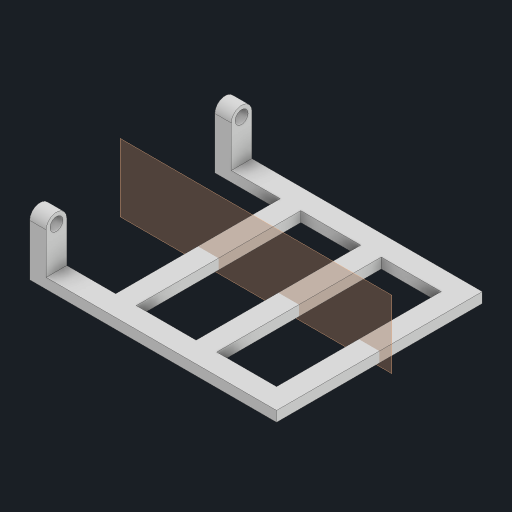
# Autodesk Inventor part: table_base
Saved by Autodesk Inventor 2024 (Build 280153000, 153)
## iProperties
Created: 2024-06-21
Part Number: table_base
Material: Generic
Document SubType Name: Modeling
Designer: mihir
Density: 1 g/cm^3
Appearance: Default
Author: mihir
Autodesk Inventor part; units mm, degrees
ref_plane "YZ Plane" through (0, 0, 0) normal (1, 0, 0) x (0, 1, 0)
ref_plane "XZ Plane" through (0, 0, 0) normal (0, 1, 0) x (-1, 0, 0)
ref_plane "XY Plane" through (0, 0, 0) normal (0, 0, 1) x (1, 0, 0)
sketch "Sketch1" plane through (0, 0, 0) normal (0, 1, 0) x (-1, 0, 0)
  line L0 (0, 0) -> (0, -100)
  line L1 (0, -100) -> (120, -100)
  line L2 (120, -100) -> (120, -90)
  line L3 (120, -90) -> (88.2057, -90)
  line L4 (88.2057, -90) -> (88.2057, -10)
  line L5 (88.2057, -10) -> (120, -10)
  line L6 (120, -10) -> (120, 0)
  line L7 (120, 0) -> (0, 0)
  line L8 (78.2057, -10) -> (49.1029, -10)
  line L9 (49.1029, -10) -> (49.1029, -90)
  line L10 (49.1029, -90) -> (78.2057, -90)
  line L11 (78.2057, -90) -> (78.2057, -10)
  line L12 (39.1029, -10) -> (10, -10)
  line L13 (10, -10) -> (10, -90)
  line L14 (10, -90) -> (39.1029, -90)
  line L15 (39.1029, -90) -> (39.1029, -10)
  dimension "d0" = 29.1029
  dimension "d1" = 120
  dimension "d2" = 10
  dimension "d3" = 100
  dimension "d4" = 10
  dimension "d5" = 10
  dimension "d6" = 10
  constraints: 32 end point, 8 perpendicular, 4 parallel, 4 point on line, 3 equal length, 2 horizontal, 1 collinear, 1 vertical
  measures "d0" distance of L13.end L14.end
  measures "d1" distance of L0.end L1.end
  measures "d2" distance of L5.end L6.end
  measures "d3" distance of L0.start L0.end
  measures "d4" distance between parallel lines of L4 L11
  measures "d5" distance between parallel lines of L0 L13
  measures "d6" distance between parallel lines of L9 L15
extrude "Extrusion1" add sketch "Sketch1" along normal blind 5
sketch "Sketch2" plane through (-120, 0, -10) normal (-1, 0, 0) x (0, 0, 1)
  line L0 (0, 0) -> (0, 5) projected
  line L1 (0, 0) -> (10, 0)
  line L2 (10, 0) -> (10, 25)
  line L3 (10, 25) -> (0, 25)
  line L4 (0, 25) -> (0, 0)
  circle A0 centre (5, 25) radius 3.15
  arc A1 (10, 25) -> (0, 25) centre (5, 25) ccw
  line L5 (10, 0) -> (10, 5) projected
  dimension "d9" = 25
  dimension "d10" = 6.3
  constraints: 8 end point, 2 centre point, 2 parallel, 2 point on circle, 1 coincident, 1 collinear, 1 horizontal, 1 midpoint, 1 perpendicular
  measures "d9" distance of L1.end L2.end
  measures "d10" diameter of A0
extrude "Extrusion2" add sketch "Sketch2" against normal blind 8
sketch "Sketch3" plane through (-112, 0, -10) normal (1, 0, 0) x (0, 0, -1)
  arc A0 (0, 25) -> (-10, 25) centre (-5, 25) ccw projected
  circle A1 centre (-5, 25) radius 3.15
  point P0 (-10, 0)
  dimension "d13" = 6.3
  constraints: 1 centre point, 1 coincident
  measures "d13" diameter of A1
extrude "Extrusion3" cut sketch "Sketch3" against normal blind 6
ref_plane "Work Plane1" through (-120, 0, -50) normal (0, 0, 1) x (1, 0, 0)
mirror "Mirror1" about plane through (-120, 0, -50) normal (0, 0, 1) of "Extrusion2", "Extrusion3"
equation "\"d1\" = table_base_length"
equation "\"d2\" = table_base_web_width"
equation "\"d3\" = table_base_width"
equation "\"d4\" = table_base_web_width"
equation "\"d5\" = table_base_web_width"
equation "\"d6\" = table_base_web_width"
equation "\"d7\" = table_base_thickness"
equation "\"d9\" = table_base_rod_height"
equation "\"d10\" = rod_diameter + rod_tolerance"
equation "\"d11\" = table_base_rod_holder_thickness"
equation "\"d13\" = rod_diameter + rod_tolerance"
equation "\"d14\" = 0.75 * table_base_rod_holder_thickness"
equation "\"table_base_length\" = 120"
equation "\"table_base_width\" = 100"
equation "\"table_base_thickness\" = 5"
equation "\"table_base_web_width\" = 10"
equation "\"table_base_rod_height\" = 25"
equation "\"rod_diameter\" = 6"
equation "\"rod_tolerance\" = 0.3"
equation "\"table_base_rod_holder_thickness\" = 8"
body "Solid1"
